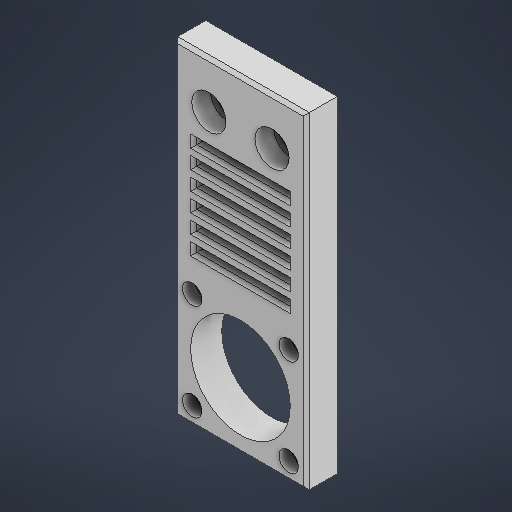
# Autodesk Inventor part: motor_cover
Saved by Autodesk Inventor 2025.1 (Build 291241000, 241)
## iProperties
Created: 2024-12-13
Part Number: motor_cover
Material: Všeobecné
Document SubType Name: Modeling
Designer: lukas
Density: 1 g/cm^3
Appearance: Výchozí
Author: lukas
Autodesk Inventor part; units mm, degrees
ref_plane "YZ Plane" through (0, 0, 0) normal (1, 0, 0) x (0, 1, 0)
ref_plane "XZ Plane" through (0, 0, 0) normal (0, 1, 0) x (-1, 0, 0)
ref_plane "XY Plane" through (0, 0, 0) normal (0, 0, 1) x (1, 0, 0)
sketch "Náčrt1" plane through (0, 0, 0) normal (0, 0, 1) x (1, 0, 0)
  line L0 (0, 29.61) -> (0, -29.61) projected
  line L1 (-29.61, 0) -> (29.61, 0) projected
  line L2 (-21.15, 21.15) -> (21.15, 21.15)
  line L3 (21.15, 21.15) -> (21.15, -21.15)
  line L4 (21.15, -21.15) -> (-21.15, -21.15)
  line L5 (-21.15, -21.15) -> (-21.15, 21.15)
  point P0 (0, 0)
  dimension "d0" = 42.3
  dimension "d1" = 42.3
  constraints: 8 end point, 2 parallel, 1 horizontal, 1 perpendicular, 2 other
  measures "d0" distance of L3.end L4.end
  measures "d1" distance of L2.end L3.end
extrude "Vysunutí1" add sketch "Náčrt1" along normal blind 10
sketch "Náčrt2" plane through (0, 0, 10) normal (0, 0, 1) x (1, 0, 0)
  line L0 (19.15, -19.15) -> (-19.15, -19.15) projected
  line L1 (19.15, 19.15) -> (19.15, -19.15) projected
  line L2 (-19.15, 19.15) -> (19.15, 19.15) projected
  line L3 (-19.15, -19.15) -> (-19.15, 19.15) projected
  point P0 (0, 0)
  point P1 (0, 0)
  constraints: 1 coincident
hole "Díra1" at (0, 0, 10) direction (0, 0, -1) diameter 32 end through all
sketch "Náčrt3" plane through (0, 0, 10) normal (0, 0, 1) x (1, 0, 0)
  circle A0 centre (0, 0) radius 16 projected
  line L0 (-29.61, 0) -> (29.61, 0) projected
  line L1 (0, -29.61) -> (0, 29.61) projected
  point P0 (-15.5, 15.5)
  point P1 (-15.5, -15.5)
  point P2 (15.5, -15.5)
  point P3 (15.5, 15.5)
  dimension "d14" = 31
  dimension "d16" = 31
  constraints: 3 symmetric about line
  measures "d14" distance of point (-15.5, 15.5) point (15.5, 15.5)
  measures "d16" distance of point (15.5, 15.5) point (15.5, -15.5)
hole "Díra2" at (-15.5, 15.5, 10) at (-15.5, -15.5, 10) at (15.5, -15.5, 10) at (15.5, 15.5, 10) direction (0, 0, -1) diameter 3.4 end through all counterbore diameter 6.3 counterbore depth 4 clearance for "Strojní šroub se zápustnou hlavou" size "M3" standard "Ansi M metrický profil"
chamfer "Zkosení2" distance 1 angle 45 3 edges at (21.15, 0, 10) (0, -21.15, 10) (-21.15, 0, 10)
sketch "Náčrt4" plane through (-21.15, 21.15, 0) normal (0, 1, 0) x (1, 0, 0)
  line L0 (1, -10) -> (0, -9) projected
  line L1 (41.3, -10) -> (1, -10) projected
  line L2 (42.3, -9) -> (41.3, -10) projected
  line L3 (42.3, 0) -> (42.3, -9) projected
  line L4 (42.3, 0) -> (0, 0) projected
  line L5 (0, 0) -> (0, -9) projected
  line L6 (0, 0) -> (42.3, 0)
  line L7 (42.3, 0) -> (42.3, -10)
  line L8 (42.3, -10) -> (0, -10)
  line L9 (0, -10) -> (0, 0)
  point P0 (21.15, 0)
  dimension "d27" = 42.3
  constraints: 8 end point, 2 parallel, 1 horizontal, 1 perpendicular, 1 point on line
  measures "d27" distance between parallel lines of L5 L7
extrude "Vysunutí2" add sketch "Náčrt4" along normal blind 62.7 contours L0 L5 L4 L3 L2 L1
chamfer "Zkosení3" distance 1 angle 45 1 edges at (0, 83.85, 10)
sketch "Náčrt5" plane through (0, 0, 10) normal (0, 0, 1) x (1, 0, 0)
  line L0 (-20.15, 82.85) -> (20.15, 82.85) projected
  line L1 (-20.15, -20.15) -> (-20.15, 82.85) projected
  line L2 (20.15, -20.15) -> (-20.15, -20.15) projected
  line L3 (20.15, -20.15) -> (20.15, 82.85) projected
  circle A0 centre (0, 0) radius 16 projected
  circle A1 centre (-15.5, 15.5) radius 3.15 projected
  circle A2 centre (-15.5, -15.5) radius 3.15 projected
  circle A3 centre (15.5, -15.5) radius 3.15 projected
  circle A4 centre (15.5, 15.5) radius 3.15 projected
  line L4 (21.15, 83.85) -> (-21.15, 83.85) projected
  point P0 (10.15, 68.85)
  dimension "d40" = 15
  dimension "d41" = 10
  measures "d40" distance from line of L4 point (10.15, 68.85)
  measures "d41" distance from line of L3 point (10.15, 68.85)
hole "Díra3" at (10.15, 68.85, 10) direction (0, 0, -1) diameter 6.6 end through all counterbore diameter 11 counterbore depth 6 clearance for "Strojní šroub se zápustnou hlavou" size "M6" standard "Ansi M metrický profil"
mirror "Zrcadlit1" about plane through (0, 0, 0) normal (1, 0, 0) of "Díra3"
sketch "Náčrt6" plane through (0, 0, 10) normal (0, 0, 1) x (1, 0, 0)
  circle A0 centre (-10.15, 68.85) radius 5.5 projected
  circle A1 centre (10.15, 68.85) radius 5.5 projected
  line L0 (-20.15, 82.85) -> (20.15, 82.85) projected
  line L1 (-20.15, -20.15) -> (-20.15, 82.85) projected
  line L2 (20.15, -20.15) -> (-20.15, -20.15) projected
  line L3 (20.15, -20.15) -> (20.15, 82.85) projected
  circle A2 centre (0, 0) radius 16 projected
  circle A3 centre (-15.5, 15.5) radius 3.15 projected
  circle A4 centre (-15.5, -15.5) radius 3.15 projected
  circle A5 centre (15.5, -15.5) radius 3.15 projected
  circle A6 centre (15.5, 15.5) radius 3.15 projected
  line L4 (-15, 58.85) -> (15, 58.85)
  line L5 (15, 58.85) -> (15, 56.85)
  line L6 (15, 56.85) -> (-15, 56.85)
  line L7 (-15, 56.85) -> (-15, 58.85)
  line L8 (0, -42.15) -> (0, 104.85) projected
  dimension "d42" = 30
  dimension "d43" = 2
  dimension "d44" = 10
  constraints: 8 end point, 2 parallel, 1 horizontal, 1 perpendicular, 1 other
  measures "d42" distance of L4.start L4.end
  measures "d43" distance between parallel lines of L4 L6
  measures "d44" distance from line of A0.centre L4
extrude "Vysunutí3" cut sketch "Náčrt6" against normal through all contours L8 L6 L7 L4 | L4 L5 L6 L8
chamfer "Zkosení4" distance 1 angle 45 4 edges at (0, 58.85, 10) (15, 57.85, 10) (0, 56.85, 10) (-15, 57.85, 10)
pattern_linear "Obdélníkové pole1" count 6 spacing 6 along (0, -1, 0) of "Vysunutí3", "Zkosení4"
